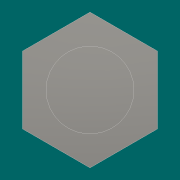
# Autodesk Inventor part: PCB SEPARADOR
Saved by Autodesk Inventor 2019 (Build 230136000, 136)
## iProperties
Created: 2023-08-26
Part Number: PCB SEPARADOR
Material: Stainless Steel
Document SubType Name: Sheet Metal
Designer: Familia CS
Density: 8 g/cm^3
Appearance: Semi-Polished
Sheet Metal Rule: Default
Author: Familia CS
Autodesk Inventor part; units mm, degrees
ref_plane "YZ Plane" through (0, 0, 0) normal (1, 0, 0) x (0, 1, 0)
ref_plane "XZ Plane" through (0, 0, 0) normal (0, 1, 0) x (-1, 0, 0)
ref_plane "XY Plane" through (0, 0, 0) normal (0, 0, 1) x (1, 0, 0)
sketch "Sketch6" plane through (0, 0, 0) normal (0, 0, 1) x (1, 0, 0)
  line L0 (0, 2.6558) -> (2.3, 1.3279)
  line L1 (2.3, 1.3279) -> (2.3, -1.3279)
  line L2 (2.3, -1.3279) -> (0, -2.6558)
  line L3 (0, -2.6558) -> (-2.3, -1.3279)
  line L4 (-2.3, -1.3279) -> (-2.3, 1.3279)
  line L5 (-2.3, 1.3279) -> (0, 2.6558)
  point P0 (0, 0)
  point P1 (0, 0)
  dimension "d15" = 4.6
  constraints: 12 end point, 1 coincident, 13 other
  measures "d15" distance between parallel lines of L1 L4
extrude "Extrusion3" add sketch "Sketch6" along normal blind 15
sketch "Sketch7" plane through (0, 0, 0) normal (0, 0, -1) x (-1, 0, 0)
  circle A0 centre (0, 0) radius 1.5
  line L0 (0, 2.6558) -> (2.3, 1.3279) projected
  line L1 (0, 2.6558) -> (2.3, 1.3279)
  line L2 (2.3, 1.3279) -> (2.3, -1.3279)
  line L3 (2.3, -1.3279) -> (0, -2.6558)
  line L4 (0, -2.6558) -> (-2.3, -1.3279)
  line L5 (-2.3, -1.3279) -> (-2.3, 1.3279)
  line L6 (-2.3, 1.3279) -> (0, 2.6558)
  dimension "d18" = 3
  constraints: 12 end point, 2 coincident, 1 centre point, 13 other
  measures "d18" diameter of A0
extrude "Extrusion4" cut sketch "Sketch7" against normal blind 6
thread "Thread2" size "M3x0.5" class "6g" standard "ISO Metric profile" full length
sketch "Sketch8" plane through (0, 0, 15) normal (0, 0, 1) x (1, 0, 0)
  circle A0 centre (0, 0) radius 1.5
  dimension "d23" = 3
  constraints: 1 centre point, 1 coincident
  measures "d23" diameter of A0
extrude "Extrusion5" cut sketch "Sketch8" against normal blind 6
thread "Thread3" size "M3x0.5" class "6H" standard "ANSI Metric M Profile" full length
equation "\"BendRadius\" = Thickness"
equation "\"BendReliefWidth\" = Thickness"
equation "\"BendReliefDepth\" = 0.5 * Thickness"
equation "\"CornerReliefSize\" = 4 * Thickness"
equation "\"MinimumRemnant\" = 2 * Thickness"
equation "\"TransitionRadius\" = BendRadius"
equation "\"JacobiRadiusSize\" = Thickness"
equation "\"GapSize\" = Thickness"
equation "\"Thickness\" = 0.5"
body "Solid2"
